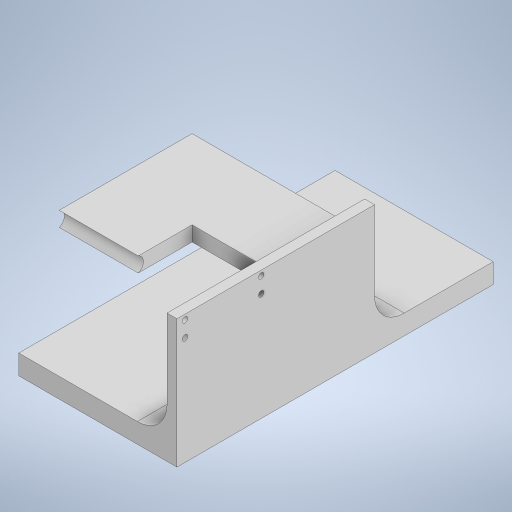
# Autodesk Inventor part: motor plate
Saved by Autodesk Inventor 2024.2 (Build 282272000, 272)
## iProperties
Created: 2024-07-10
Part Number: motor plate
Material: Generic
Document SubType Name: Modeling
Designer: Tom
Density: 1 g/cm^3
Appearance: Default
Author: Tom
Autodesk Inventor part; units mm, degrees
ref_plane "YZ Plane" through (0, 0, 0) normal (1, 0, 0) x (0, 1, 0)
ref_plane "XZ Plane" through (0, 0, 0) normal (0, 1, 0) x (-1, 0, 0)
ref_plane "XY Plane" through (0, 0, 0) normal (0, 0, 1) x (1, 0, 0)
sketch "Sketch1" plane through (0, 0, 0) normal (1, 0, 0) x (0, 1, 0)
  line L0 (0, 0) -> (19.05, 0)
  line L1 (19.05, 0) -> (19.05, -127)
  line L2 (19.05, -127) -> (0, -127)
  line L3 (0, -127) -> (0, 0)
  dimension "d0" = 19.05
  dimension "d1" = 127
  constraints: 8 end point, 2 parallel, 1 horizontal, 1 perpendicular
  measures "d0" distance of L0.start L0.end
  measures "d1" distance of L0.end L1.end
extrude "Extrusion1" add sketch "Sketch1" along normal blind 6.35
sketch "Sketch2" plane through (6.35, 0, 0) normal (1, 0, 0) x (0, 0, -1)
  circle A0 centre (5.1751, 15.875) radius 1.7526
  circle A1 centre (5.1751, 5.875) radius 1.7526
  line L0 (127, 19.05) -> (0, 19.05) projected
  circle A2 centre (54.1717, 15.875) radius 1.7526
  circle A3 centre (54.1717, 5.875) radius 1.7526
  point P0 (0, 0)
  dimension "d4" = 3.5052
  dimension "d5" = 3.5052
  dimension "d6" = 10
  dimension "d7" = 3.175
  dimension "d11" = 3.5052
  dimension "d12" = 48.9966
  dimension "d13" = 3.5052
  constraints: 4 centre point
  measures "d4" diameter of A0
  measures "d5" diameter of A1
  measures "d6" distance of A1.centre A0.centre
  measures "d7" distance from line of L0 A0.centre
  measures "d11" diameter of A2
  measures "d12" distance of A0.centre A2.centre
  measures "d13" diameter of A3
extrude "Extrusion2" cut sketch "Sketch2" against normal through all
sketch "Sketch3" plane through (0, 0, -127) normal (0, -1, 0) x (1, 0, 0)
  line L0 (6.35, 0) -> (6.35, 127) projected
  line L1 (0, 0) -> (0, 127) projected
  line L2 (6.35, 127) -> (0, 127)
  line L3 (0, 127) -> (0, 0)
  line L4 (0, 0) -> (6.35, 0)
  line L5 (6.35, 0) -> (6.35, 127)
  point P0 (0, 127)
  constraints: 8 end point, 2 parallel, 1 horizontal, 1 perpendicular
extrude "Extrusion3" add sketch "Sketch3" along normal blind 50.8
sketch "Sketch4" plane through (0, -50.8, -127) normal (0, -1, 0) x (1, 0, 0)
  line L0 (6.35, 0) -> (6.35, 127) projected
  line L1 (6.35, 127) -> (-95.25, 127)
  line L2 (-95.25, 127) -> (-95.25, -76.2)
  line L3 (-95.25, -76.2) -> (6.35, -76.2)
  line L4 (6.35, -76.2) -> (6.35, 127)
  point P0 (0, 127)
  point P1 (6.35, 0)
  dimension "d16" = 203.2
  dimension "d17" = 101.6
  constraints: 8 end point, 2 parallel, 1 horizontal, 1 perpendicular
  measures "d16" distance of L3.end L0.end
  measures "d17" distance of L0.end L1.end
extrude "Extrusion4" add sketch "Sketch4" along normal blind 12.7
fillet "Fillet1" radius 19.05 1 edges at (0, -50.8, -63.5)
fillet "Fillet2" radius 19.05 2 edges at (-9.525, -50.8, -127) (3.175, -50.8, -127)
sketch "Sketch5" plane through (0, 0, 0) normal (-1, 0, 0) x (0, 0, 1)
  line L0 (-111.3217, 15.6337) -> (-60.5217, 15.6337)
  line L1 (-60.5217, 15.6337) -> (-60.5217, 6.1087)
  line L2 (-60.5217, 6.1087) -> (-111.3217, 6.1087)
  line L3 (-111.3217, 6.1087) -> (-111.3217, 15.6337)
  circle A0 centre (-54.1717, 5.875) radius 1.7526 projected
  circle A1 centre (-54.1717, 15.875) radius 1.7526 projected
  point P0 (0, 0)
  point P1 (-60.5217, 10.8712)
  dimension "d22" = 9.525
  dimension "d23" = 50.8
  dimension "d26" = 5.0038
  dimension "d27" = 6.35
  constraints: 8 end point, 2 parallel, 1 horizontal, 1 midpoint, 1 perpendicular
  measures "d22" distance of L2.end L0.start
  measures "d23" distance of L0.start L0.end
  measures "d26" vertical distance of A1.centre point (-60.522, 10.871)
  measures "d27" distance from line of A1.centre L1
extrude "Extrusion5" add sketch "Sketch5" along normal blind 95.25 contours L0 L1 L2 L3
sketch "Sketch6" plane through (0, 6.1087, -60.5217) normal (0, 0, 1) x (1, 0, 0)
  line L0 (0, 9.525) -> (-95.25, 9.525) projected
  line L1 (0, 0) -> (-95.25, 0) projected
  line L2 (-95.25, 9.525) -> (-44.45, 9.525)
  line L3 (-44.45, 9.525) -> (-44.45, 0)
  line L4 (-44.45, 0) -> (-95.25, 0)
  line L5 (-95.25, 0) -> (-95.25, 9.525)
  point P0 (0, -6.1087)
  dimension "d30" = 50.8
  constraints: 8 end point, 2 parallel, 1 horizontal, 1 perpendicular, 1 point on line
  measures "d30" distance between parallel lines of L5 L3
extrude "Extrusion6" add sketch "Sketch6" along normal blind 38.1
sketch "Sketch7" plane through (-95.25, 0, 0) normal (-1, 0, 0) x (0, 0, 1)
  line L0 (-22.4217, 15.6337) -> (-22.4217, 6.1087) projected
  arc A0 (-22.4217, 15.6337) -> (-22.4217, 6.1087) centre (-24.1894, 10.8712) ccw
  line L1 (-22.4217, 15.6337) -> (-22.4217, 6.1087)
  point P0 (0, 0)
  dimension "d33" = 5.08
  constraints: 2 end point, 2 point on circle, 1 centre point, 1 vertical
  measures "d33" radius of A0
extrude "Extrusion7" cut sketch "Sketch7" against normal up to surface (50.8 mm away)
body "Solid1"
